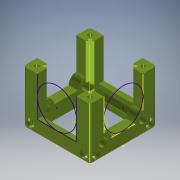
# Autodesk Inventor part: 10_Cube_v0
Saved by Autodesk Inventor 2019 (Build 230136000, 136)
## iProperties
Created: 2018-05-19
Part Number: 10_Cube_v0
Material: Generisch
Document SubType Name: Modeling
Designer: diederichbenedict
Density: 1 g/cm^3
Appearance: IPHT_Grün
Mass: 20.3218 g
Surface Area: 129.075 cm^2
Volume: 20.3218 cm^3
Author: diederichbenedict
Autodesk Inventor part; units mm, degrees
ref_plane "YZ Plane" through (0, 0, 0) normal (1, 0, 0) x (0, 1, 0)
ref_plane "XZ Plane" through (0, 0, 0) normal (0, 1, 0) x (-1, 0, 0)
sketch "Skizze1" plane through (0, 0, 0) normal (0, 0, 1) x (1, 0, 0)
  line L0 (-24.9, 24.9) -> (24.9, 24.9)
  line L1 (24.9, 24.9) -> (24.9, -24.9)
  line L2 (24.9, -24.9) -> (-24.9, -24.9)
  line L3 (-24.9, -24.9) -> (-24.9, 24.9)
  line L4 (-24.9, 24.9) -> (24.9, -24.9) construction
  line L5 (24.9, 24.9) -> (-24.9, -24.9) construction
  line L6 (14.6269, -17.9) -> (-14.6269, -17.9)
  line L7 (-17.9, -14.6269) -> (-17.9, 14.6269)
  line L8 (-14.6269, 17.9) -> (14.6269, 17.9)
  line L9 (17.9, 14.6269) -> (17.9, -14.6269)
  line L10 (20.5, -20.5) -> (-20.5, 20.5) construction
  line L11 (-20.5, -20.5) -> (20.5, 20.5) construction
  line L12 (-14.6269, 17.9) -> (-17.9, 14.6269)
  line L13 (-14.6269, 17.9) -> (-9.9981, 17.9) construction
  line L14 (17.9, -14.6269) -> (14.6269, -17.9)
  line L15 (17.9, -14.6269) -> (22.5288, -14.6269) construction
  line L16 (-17.9, -14.6269) -> (-14.6269, -17.9)
  line L17 (14.6269, 17.9) -> (17.9, 14.6269)
  point P0 (0, 0)
  dimension "d0" = 49.8
  dimension "d1" = 49.8
  dimension "d2" = 41
  dimension "d3" = 41
  dimension "d4" = 135
  dimension "d5" = 23
  dimension "d6" = 135
  dimension "d7" = 23
  dimension "a1" = 23
  dimension "d9" = 23
  dimension "a2" = 7
  dimension "d42" = 7
  dimension "d43" = 7
  dimension "d44" = 7
  constraints: 36 end point, 4 horizontal, 4 midpoint, 4 parallel, 4 perpendicular, 2 equal length
  measures "d0" distance of L1.end L2.end
  measures "d1" distance of L0.end L1.end
  measures "d2" distance of L10.end L11.end
  measures "d3" distance of L11.start L10.end
  measures "d4" angle of L12 L13
  measures "d5" distance from line of point (0, 0) L12
  measures "d6" angle of L14 L15
  measures "d7" distance from line of point (0, 0) L14
  measures "a1" distance from line of point (0, 0) L17
  measures "d9" distance from line of L16 point (0, 0)
  measures "a2" distance between parallel lines of L8 L0
  measures "d42" distance between parallel lines of L3 L7
  measures "d43" distance between parallel lines of L2 L6
  measures "d44" distance between parallel lines of L1 L9
extrude "Extrusion1" add sketch "Skizze1" along normal blind 10.3
sketch "Skizze2" plane through (0, 0, 10.3) normal (0, 0, 1) x (1, 0, 0)
  line L0 (-17.9, 14.6269) -> (-14.6269, 17.9) construction
  line L1 (-14.6269, 17.9) -> (14.6269, 17.9) construction
  line L2 (14.6269, 17.9) -> (17.9, 14.6269) construction
  line L3 (17.9, 14.6269) -> (17.9, -14.6269) construction
  line L4 (17.9, -14.6269) -> (14.6269, -17.9) construction
  line L5 (14.6269, -17.9) -> (-14.6269, -17.9) construction
  line L6 (-14.6269, -17.9) -> (-17.9, -14.6269) construction
  line L7 (-17.9, -14.6269) -> (-17.9, 14.6269) construction
  line L8 (24.9, 24.9) -> (-24.9, 24.9) construction
  line L9 (-24.9, 24.9) -> (-24.9, -24.9) construction
  line L10 (-24.9, -24.9) -> (24.9, -24.9) construction
  line L11 (24.9, -24.9) -> (24.9, 24.9) construction
  line L12 (-17.9, -14.6269) -> (-24.9, -14.6269)
  line L13 (-24.9, -24.9) -> (-24.9, 24.9) projected
  line L14 (-24.9, -14.6269) -> (-24.9, -24.9)
  line L15 (-17.9, -14.6269) -> (-14.6269, -17.9) projected
  line L16 (-17.9, -14.6269) -> (-14.6269, -17.9)
  line L17 (-14.6269, -17.9) -> (-14.6269, -24.9)
  line L18 (24.9, -24.9) -> (-24.9, -24.9) projected
  line L19 (-24.9, -24.9) -> (-14.6269, -24.9)
  line L20 (-17.9, -14.9) -> (-17.9, 14.9) projected
  line L21 (14.9, -17.9) -> (-14.9, -17.9) projected
  line L22 (17.9, 14.9) -> (17.9, -14.9) projected
  line L23 (-14.9, 17.9) -> (-9.9, 17.9) projected
  circle A0 centre (0, 0) radius 17.9
  line L24 (14.6269, -17.9) -> (17.9, -14.6269)
  line L25 (17.9, -14.6269) -> (24.9, -14.6269)
  line L26 (24.9, -24.9) -> (24.9, -14.6269)
  line L27 (14.6269, -24.9) -> (24.9, -24.9)
  line L28 (14.6269, -17.9) -> (14.6269, -24.9)
  line L29 (17.9, 14.6269) -> (14.6269, 17.9)
  line L30 (14.6269, 17.9) -> (14.6269, 24.9)
  line L31 (24.9, 24.9) -> (14.6269, 24.9)
  line L32 (24.9, 14.6269) -> (24.9, 24.9)
  line L33 (17.9, 14.6269) -> (24.9, 14.6269)
  line L34 (-14.6269, 17.9) -> (-17.9, 14.6269)
  line L35 (-17.9, 14.6269) -> (-24.9, 14.6269)
  line L36 (-24.9, 24.9) -> (-24.9, 14.6269)
  line L37 (-14.6269, 24.9) -> (-24.9, 24.9)
  line L38 (-14.6269, 17.9) -> (-14.6269, 24.9)
  line L39 (0, 0) -> (24.9, -24.9) construction
  line L40 (14.4957, -15.9099) -> (16.617, -18.0312)
  line L41 (16.617, -18.0312) -> (18.0312, -16.617)
  line L42 (18.0312, -16.617) -> (15.9099, -14.4957)
  line L43 (15.9099, -14.4957) -> (14.4957, -15.9099)
  line L44 (14.4957, -15.9099) -> (18.0312, -16.617) construction
  line L45 (16.617, -18.0312) -> (15.9099, -14.4957) construction
  line L46 (14.6269, -17.9) -> (17.9, -14.6269) projected
  point P0 (16.2635, -16.2635)
  point P1 (16.9706, -15.5563)
  point P2 (15.5563, -16.9706)
  dimension "d80" = 360
  dimension "d101" = 3
  dimension "d102" = 2
  constraints: 54 end point, 6 point on line, 5 midpoint, 3 perpendicular, 3 tangent, 2 collinear, 2 parallel, 1 centre point, 1 vertical, 41 other
  measures "d101" distance of L40.start L40.end
  measures "d102" distance of L41.end L40.end
extrude "Extrusion2" add sketch "Skizze2" along normal blind 29.4 contours L15 L17 L18 L13 L12 | L29 L30 L31 L32 L33 | L13 L37 L38 L34 L35 | L28 L24 L40 L41 L42 L25 L26 L18 | L24 L42 L41 L40
fillet "Rundung1" radius 2 8 edges at (24.9, 24.9, 19.85) (24.9, 0, 0) (24.9, -24.9, 19.85) (-24.9, 24.9, 19.85) (-24.9, -24.9, 19.85) (-24.9, 0, 0) (0, -24.9, 0) (0, 24.9, 0)
sketch "Skizze3" plane through (0, 0, 39.7) normal (0, 0, 1) x (1, 0, 0)
  line L0 (20, 20) -> (-20, 20) construction
  line L1 (-20, 20) -> (-20, -20) construction
  line L2 (-20, -20) -> (20, -20) construction
  line L3 (20, -20) -> (20, 20) construction
  line L4 (20, 20) -> (-20, -20) construction
  line L5 (-20, 20) -> (20, -20) construction
  line L6 (22.9, -22.9) -> (20.7681, -22.9) projected
  line L7 (22.9, -20.7681) -> (22.9, -22.9) projected
  arc A0 (20.7681, -22.9) -> (22.9, -20.7681) centre (20, -20) ccw projected
  point P0 (0, 0)
  point P1 (-20, 20)
  point P2 (20, -20)
  point P3 (20, -20)
  point P4 (20, -20)
  point P5 (-20, -20)
  point P6 (-20, -20)
  point P7 (-15.7881, 5.2)
  point P8 (-15.7881, -5.2)
  dimension "d15" = 40
  dimension "d16" = 40
  constraints: 12 end point, 2 midpoint, 2 parallel, 1 horizontal, 1 perpendicular
  measures "d15" distance of L2.end L1.end
  measures "d16" distance of L1.end L0.end
hole "Bohrung1" at (20, -20, 39.7) at (-20, -20, 39.7) at (-20, 20, 39.7) at (20, 20, 39.7) direction (0, 0, -1) diameter 2.9 depth 10 tip angle 118
sketch "Skizze4" plane through (0, 0, 0) normal (0, 0, -1) x (-1, 0, 0)
  circle A0 centre (20, -20) radius 1.45 projected
  circle A1 centre (20, 20) radius 1.45 projected
  line L0 (14.6269, 17.9) -> (17.9, 14.6269) projected
  line L1 (17.9, 14.6269) -> (17.9, -14.6269) projected
  line L2 (17.9, -14.6269) -> (14.6269, -17.9) projected
  line L3 (14.6269, -17.9) -> (-14.6269, -17.9) projected
  line L4 (-14.6269, -17.9) -> (-17.9, -14.6269) projected
  line L5 (-17.9, -14.6269) -> (-17.9, 14.6269) projected
  line L6 (-17.9, 14.6269) -> (-14.6269, 17.9) projected
  line L7 (-14.6269, 17.9) -> (14.6269, 17.9) projected
  line L8 (-22.9, 22.9) -> (22.9, 22.9) projected
  line L9 (-22.9, -22.9) -> (-22.9, 22.9) projected
  line L10 (22.9, -22.9) -> (-22.9, -22.9) projected
  line L11 (22.9, 22.9) -> (22.9, -22.9) projected
  circle A2 centre (-20, -20) radius 1.45 projected
  circle A3 centre (-20, 20) radius 1.45 projected
  point P0 (0, 0)
  point P1 (19.8136, -18.5116)
  point P2 (18.5116, -19.8136)
  point P3 (18.5116, 19.8136)
  point P4 (19.8136, 18.5116)
  point P5 (-18.5116, -19.8136)
  point P6 (-19.8136, -18.5116)
  point P7 (-19.8136, 18.5116)
  point P8 (-18.5116, 19.8136)
  constraints: 6 other
hole "Bohrung2" at (-20, -20, 0) at (-20, 20, 0) at (20, -20, 0) at (20, 20, 0) direction (0, 0, 1) diameter 3 depth 15 tip angle 118 counterbore diameter 6.2 counterbore depth 2.5
sketch "Skizze8" plane through (24.9, -14.6269, 10.3) normal (1, 0, 0) x (0, 0, -1)
  line L0 (-39.7, 33.8588) -> (-39.7, -4.605) projected
  arc A0 (-37.7, 39.5269) -> (-39.7, 37.5269) centre (-37.7, 37.5269) ccw projected
  arc A1 (8.3, -10.2731) -> (10.3, -8.2731) centre (8.3, -8.2731) ccw projected
  arc A2 (-39.7, -8.2731) -> (-37.7, -10.2731) centre (-37.7, -8.2731) ccw projected
  arc A3 (10.3, 37.5269) -> (8.3, 39.5269) centre (8.3, 37.5269) ccw projected
  line L1 (-37.7, -8.2731) -> (8.3, 37.5269) construction
  line L2 (8.3, -8.2731) -> (8.3, 37.5269) construction
  line L3 (8.3, -8.2731) -> (-37.7, 37.5269) construction
  circle A4 centre (-14.7, 14.6269) radius 6.587 construction
  line L4 (-34.7, -5.3731) -> (5.3, -5.3731) construction
  line L5 (5.3, -5.3731) -> (5.3, 34.6269) construction
  line L6 (5.3, 34.6269) -> (-34.7, 34.6269) construction
  line L7 (-34.7, 34.6269) -> (-34.7, -5.3731) construction
  line L8 (-34.7, -5.3731) -> (5.3, 34.6269) construction
  line L9 (5.3, -5.3731) -> (-34.7, 34.6269) construction
  point P0 (10.3, 14.6269)
  dimension "d110" = 40
  dimension "d111" = 40
  constraints: 16 end point, 3 midpoint, 2 parallel, 1 centre point, 1 horizontal, 1 perpendicular
  measures "d110" distance of L6.end L5.end
  measures "d111" distance of L5.end L4.end
sketch "Skizze9" plane through (14.6269, 17.9, 10.3) normal (-1, 0, 0) x (0, 0, 1)
  line L0 (-3.2288, -37.966) -> (32.6288, -37.966) construction
  line L1 (32.6288, -37.966) -> (34.766, -35.8288) construction
  line L2 (34.766, -35.8288) -> (34.766, 0.0288) construction
  line L3 (34.766, 0.0288) -> (32.6288, 2.166) construction
  line L4 (32.6288, 2.166) -> (-3.2288, 2.166) construction
  line L5 (-3.2288, 2.166) -> (-5.366, 0.0288) construction
  line L6 (-5.366, 0.0288) -> (-5.366, -35.8288) construction
  line L7 (-5.366, -35.8288) -> (-3.2288, -37.966) construction
  circle A0 centre (29.7, -2.9) radius 3.2639 construction
  circle A1 centre (-0.3, -2.9) radius 3.2639 construction
  circle A2 centre (-0.3, -32.9) radius 3.2639 construction
  circle A3 centre (29.7, -32.9) radius 3.2639 construction
  circle A4 centre (14.7, -17.9) radius 13.3985 construction
  line L8 (-3.643, 3.166) -> (33.043, 3.166)
  line L9 (33.043, 3.166) -> (35.766, 0.443)
  line L10 (35.766, 0.443) -> (35.766, -36.243)
  line L11 (35.766, -36.243) -> (33.043, -38.966)
  line L12 (33.043, -38.966) -> (-3.643, -38.966)
  line L13 (-3.643, -38.966) -> (-6.366, -36.243)
  line L14 (-6.366, -36.243) -> (-6.366, 0.443)
  line L15 (-6.366, 0.443) -> (-3.643, 3.166)
  point P0 (-10.3, -17.9)
  dimension "d82" = 1
  constraints: 16 end point, 7 other
  measures "d82" distance between parallel lines of L4 L8
extrude "Extrusion5" cut sketch "Skizze9" along normal up to surface (29.2538 mm away)
sketch "Skizze10" plane through (-24.9, -14.6269, 10.3) normal (-1, 0, 0) x (0, 0, 1)
  circle A0 centre (-0.3, 29.6269) radius 3.2639 construction
  circle A1 centre (-0.3, -0.3731) radius 3.2639 construction
  circle A2 centre (29.7, 29.6269) radius 3.2639 construction
  circle A3 centre (29.7, -0.3731) radius 3.2639 construction
  circle A4 centre (29.7, 29.6269) radius 3.3139
  circle A5 centre (29.7, -0.3731) radius 3.3139
  line L0 (-8.3, -10.2731) -> (29.4, -10.2731) projected
  line L1 (29.4, 39.5269) -> (-8.3, 39.5269) projected
  circle A6 centre (-0.3, -0.3731) radius 2.95
  circle A7 centre (-0.3, 29.6269) radius 2.95
  point P0 (-10.3, 14.6269)
  dimension "a4" = 0.05
  dimension "d90" = 0.05
  dimension "d130" = 9.9
  dimension "d131" = 9.9
  dimension "d132" = 5.9
  dimension "d133" = 5.9
  constraints: 4 centre point, 2 coincident
  measures "a4" radial gap between concentric circles of A2 A4
  measures "d90" radial gap between concentric circles of A3 A5
  measures "d130" distance from line of L0 A1.centre
  measures "d131" distance from line of L1 A0.centre
  measures "d132" diameter of A6
  measures "d133" diameter of A7
extrude "Extrusion6" cut sketch "Skizze10" against normal through all contours A6 | A7
sketch "Skizze11" plane through (-24.9, -22.9, 2) normal (-1, 0, 0) x (0, 0, 1)
  line L0 (10.9263, 37.5269) -> (37.7, 37.5269) construction
  line L1 (37.7, 45.8) -> (37.7, 37.5269) construction
  line L2 (0, 45.8) -> (37.7, 45.8) construction
  line L3 (0, 0) -> (0, 45.8) construction
  line L4 (37.7, 0) -> (0, 0) construction
  line L5 (37.7, 8.2731) -> (37.7, 0) construction
  line L6 (10.9263, 8.2731) -> (37.7, 8.2731) construction
  line L7 (8.3, 34.9653) -> (8.3, 10.8347) construction
  arc A0 (8.3, 34.7503) -> (11.1419, 37.5269) centre (8.1696, 37.7265) ccw
  line L8 (10.9263, 8.2731) -> (37.7, 8.2731) projected
  line L9 (8.3, 10.8347) -> (8.3, 34.7503) projected
  arc A1 (11.1419, 8.2731) -> (8.3, 11.0497) centre (8.1696, 8.0735) ccw
  line L10 (8.1696, 8.0735) -> (14.1696, 8.0735) construction
  line L11 (14.1696, 8.0735) -> (14.1696, 14.0735) construction
  line L12 (14.1696, 14.0735) -> (8.1696, 14.0735) construction
  line L13 (8.1696, 14.0735) -> (8.1696, 8.0735) construction
  line L14 (8.1696, 37.7265) -> (14.1696, 37.7265) construction
  line L15 (14.1696, 37.7265) -> (14.1696, 31.7265) construction
  line L16 (14.1696, 31.7265) -> (8.1696, 31.7265) construction
  line L17 (8.1696, 31.7265) -> (8.1696, 37.7265) construction
  arc A2 (8.3, 31.7265) -> (14.1696, 37.5269) centre (8, 37.9) ccw
  arc A3 (14.1696, 8.2731) -> (8.3, 14.0735) centre (8, 7.9) ccw
  line L18 (11.1419, 37.5269) -> (37.7, 37.5269) projected
  line L19 (14.1696, 37.5269) -> (11.1419, 37.5269)
  line L20 (8.3, 34.7503) -> (8.3, 31.7265)
  line L21 (8.3, 14.0735) -> (8.3, 11.0497)
  line L22 (11.1419, 8.2731) -> (14.1696, 8.2731)
  arc A4 (8.3, 10.8347) -> (10.9263, 8.2731) centre (8, 7.9) ccw projected
  arc A5 (10.9263, 37.5269) -> (8.3, 34.9653) centre (8, 37.9) ccw projected
  dimension "d124" = 6
  dimension "d125" = 6
  dimension "d126" = 6
  dimension "d127" = 6
  constraints: 24 end point, 8 point on circle, 8 point on line, 5 parallel, 4 centre point, 3 perpendicular, 2 collinear, 2 horizontal
  measures "d124" distance of L12.end L11.end
  measures "d125" distance of L11.end L10.end
  measures "d126" distance of L15.end L16.end
  measures "d127" distance of L14.end L15.end
extrude "Extrusion7" add sketch "Skizze11" against normal up to surface (7 mm away) contours A3 L8 A1 L9 | A0 L18 A2 L9
sketch "Skizze12" plane through (24.9, -22.9, 2) normal (1, 0, 0) x (0, 0, -1)
  arc A0 (-8.3, 14.0735) -> (-14.1696, 8.2731) centre (-8, 7.9) ccw projected
  arc A1 (-14.1696, 37.5269) -> (-8.3, 31.7265) centre (-8, 37.9) ccw projected
  arc A2 (-11.1419, 37.5269) -> (-8.3, 34.7503) centre (-8.1696, 37.7265) ccw projected
  arc A3 (-8.3, 11.0497) -> (-11.1419, 8.2731) centre (-8.1696, 8.0735) ccw projected
  line L0 (-8.3, 8.2731) -> (-37.7, 8.2731) projected
  line L1 (-14.1696, 8.2731) -> (-11.1419, 8.2731)
  line L2 (-8.3, 11.0497) -> (-8.3, 14.0735)
  line L3 (-8.3, 37.5269) -> (-8.3, 8.2731) projected
  line L4 (-8.3, 34.7503) -> (-8.3, 31.7265)
  line L5 (-14.1696, 37.5269) -> (-11.1419, 37.5269)
  constraints: 8 end point, 2 collinear, 1 perpendicular, 1 vertical
ref_plane "Arbeitsebene1" through (17.9, -21.066, 43) normal (-1, 0, 0) x (0, 0, 1)
extrude "Extrusion8" add sketch "Skizze12" against normal up to surface (7 mm away) contours L2 A3 L0 A0 | A1 L5 A2 L3
sketch "Skizze13" plane through (0, 0, 39.7) normal (0, 0, 1) x (1, 0, 0)
  arc A0 (22.9, -24.9) -> (24.9, -22.9) centre (22.9, -22.9) ccw construction
  line L0 (17.9, -14.6269) -> (14.6269, -17.9) construction
  line L1 (14.6269, -17.9) -> (14.6269, -24.9) construction
  line L2 (14.6269, -24.9) -> (22.9, -24.9) construction
  line L3 (16.9706, -18.3848) -> (-18.3848, 16.9706)
  line L4 (-18.3848, 16.9706) -> (-16.9706, 18.3848)
  line L5 (-16.9706, 18.3848) -> (18.3848, -16.9706)
  line L6 (18.3848, -16.9706) -> (16.9706, -18.3848)
  line L7 (16.9706, -18.3848) -> (-16.9706, 18.3848) construction
  line L8 (-18.3848, 16.9706) -> (18.3848, -16.9706) construction
  line L9 (16.9706, -18.3848) -> (66.9706, -18.3848) construction
  line L10 (18.3848, 16.9706) -> (-16.9706, -18.3848)
  line L11 (-16.9706, -18.3848) -> (-18.3848, -16.9706)
  line L12 (-18.3848, -16.9706) -> (16.9706, 18.3848)
  line L13 (16.9706, 18.3848) -> (18.3848, 16.9706)
  line L14 (18.3848, 16.9706) -> (-18.3848, -16.9706) construction
  line L15 (-16.9706, -18.3848) -> (16.9706, 18.3848) construction
  line L16 (24.9, -22.9) -> (24.9, -14.6269) projected
  line L17 (24.9, -14.6269) -> (17.9, -14.6269) projected
  line L18 (22.9, -22.9) -> (20.7681, -22.9) projected
  line L19 (22.9, -20.7681) -> (22.9, -22.9) projected
  arc A1 (20.7681, -22.9) -> (22.9, -20.7681) centre (20, -20) ccw projected
  point P0 (0, 0)
  point P1 (20, -20)
  point P2 (20, -20)
  point P3 (-20, -20)
  point P4 (20, -20)
  point P5 (-20, -20)
  point P6 (-20, -20)
  point P7 (-20, -20)
  point P8 (-15.7881, 5.2)
  point P9 (-15.7881, -5.2)
  dimension "d103" = 50
  dimension "d104" = 135
  dimension "d105" = 2
  dimension "d106" = 50
  dimension "d107" = 2
  constraints: 26 end point, 5 parallel, 4 midpoint, 2 perpendicular, 1 equal length, 1 horizontal
  measures "d103" distance of L3.start L3.end
  measures "d104" angle of L9 L3
  measures "d105" distance of L3.end L4.end
  measures "d106" distance of L10.start L10.end
  measures "d107" distance of L10.end L11.end
extrude "Extrusion9" cut sketch "Skizze13" against normal up to surface (29.4 mm away) contours L3 L10 L5 L6 | L10 L11 L12 L3 | L3 L12 L5 L10 | L3 L4 L5 L12 | L5 L12 L13 L10
hole "Bohrung3" at (24.9, -20, 5) at (24.9, 20, 5) at (24.9, -20, 45) at (24.9, 20, 45) direction (-1, 0, 0) diameter 3 depth 15 tip angle 118 counterbore diameter 6.2 counterbore depth 2.5
sketch "Skizze14" plane through (0, 0, 0) normal (0, 0, -1) x (-1, 0, 0)
  circle A0 centre (0, 0) radius 9.428
  constraints: 1 centre point, 1 coincident
pattern_circular "Runde Anordnung2" count 4 over 360 about axis through (0, 0, 0) along (0, 0, 1) of "Bohrung3"
sketch "Sketch15" plane through (24.9, 14.6269, 39.7) normal (1, 0, 0) x (0, 0, -1)
  line L0 (23.5304, 0) -> (0, 0) projected
  line L1 (29.4, -23.4534) -> (29.4, -5.8005) projected
  line L2 (23.5304, -29.2538) -> (0, -29.2538) projected
  circle A0 centre (14.7731, -14.6269) radius 14.6269
  point P0 (39.7, -14.6269)
  constraints: 3 tangent, 1 centre point
sketch "Sketch16" plane through (-14.6269, -24.9, 10.3) normal (0, -1, 0) x (1, 0, 0)
  line L0 (29.2538, 0) -> (29.2538, 29.4)
  line L1 (29.2538, 0) -> (0, 0)
  line L2 (0, 0) -> (0, 29.4)
  circle A0 centre (14.6269, 14.6269) radius 14.6269
  point P0 (14.6269, -10.3)
  constraints: 6 end point, 3 tangent, 2 vertical, 1 centre point, 1 horizontal, 4 other
equation "\"d5\" = a1"
equation "\"d7\" = a1"
equation "\"d9\" = a1"
equation "\"d42\" = a2"
equation "\"d43\" = a2"
equation "\"d44\" = a2"
equation "\"d90\" = a4"
